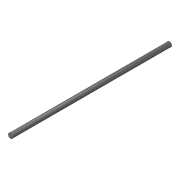
# Autodesk Inventor part: 200-60-DIFFERENTIAL-BAR-02
Saved by Autodesk Inventor 2018.2 (Build 222227000, 227)
## iProperties
Manager: feesmrt
Company: FRANC0R
Created: 2017-12-05
Part Number: 200-60-DIFFERENTIAL-BAR-02
Material: Edelstahl
Document SubType Name: Modeling
Designer: feesmrt
Density: 8 g/cm^3
Appearance: Halbpoliert
Project: Rescue Robot
Cost Center: -
Engineer: feesmrt
Authority: feesmrt
Description: Differential Long Connector Bar
Stock Number: 200-60-DIFFERENTIAL-BAR-02
Author: feesmrt
Subject: Rescue Robot
Title: Differential Long Connector Bar
Revision Number: 1
Autodesk Inventor part; units mm, degrees
ref_plane "YZ Plane" through (0, 0, 0) normal (1, 0, 0) x (0, 1, 0)
ref_plane "XZ Plane" through (0, 0, 0) normal (0, 1, 0) x (-1, 0, 0)
ref_plane "XY Plane" through (0, 0, 0) normal (0, 0, 1) x (1, 0, 0)
sketch "Skizze2" plane through (0, 0, 0) normal (0, 1, 0) x (-1, 0, 0)
  line L0 (0, -4.2) -> (0, 4.2) construction
  line L1 (-4.2, 0) -> (4.2, 0) construction
  circle A0 centre (0, 0) radius 3
  dimension "d5" = 6
  constraints: 1 centre point, 1 coincident
  measures "d5" diameter of A0
extrude "Grundkörper" add sketch "Skizze2" along normal mid plane 200
thread "M6" size "M6x1" class "6g" standard "ANSI Metric M Profile" full length
chamfer "Fase1" distance 0.5 angle 45 2 edges at (3, -100, 0) (3, 100, 0)
